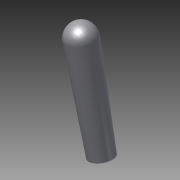
# Autodesk Inventor part: M20S3-toggles
Saved by Autodesk Inventor 2014 (Build 180170000, 170)
## iProperties
Category: PARTsolutions
Company: NKKSWITCHES
Created: 2013-12-29
Part Number: M20S3-toggles
Catalog Web Link: www.cadenas.de
Description: Bushing Mount Miniature Toggles - toggles-Series M - Miniature Toggles
Vendor: NKKSWITCHES
Document SubType Name: Modeling
Designer: PARTuser1
Manufacturer: NKKSWITCHES
Density: 1 g/cm^3
Material: Generic
Appearance: RGB(192.00000375509219,192.00000375509219,192.00000375509219)
PSOL_IDENT_0: {$CADENAS_DATA\23d-libs\nkkswitches\toggle\m\parts\m_bt_toggle.prj},217 {VTYP=3D},{NB=M20S3-toggles}
PSOL_IDENT_1: ,{LINA=M20S3-toggles},{NN=Bushing Mount Miniature Toggles - toggles},{DATE=28.05.2013 12:02:29},{GEO
PSOL_IDENT_2: MDATE=28.05.2013 14:02:00},{VERSION=},{LINEID=10},{LINESUBID=-1},{WBVAR=TGGLS,CPS,CCLR}  {NB=M20S3-t
PSOL_IDENT_3: oggles},{LINA=M20S3-toggles},{KT=DUMMY},{PN=M20S3},{SRS=M20},{TGGLSALG='S', 'S - .413\" (10.5mm) Bat
PSOL_IDENT_4: ','S2', 'S2 - .200\" (5.08mm) Bat','S3', 'S3 - .256\" (6.5mm) Bat','E', 'E - .450\" (11.4mm) Flatted
PSOL_IDENT_5: ','E2', 'E2 - .256\" (6.5mm) Flatted','E4', 'E4 - .840\" (21.3mm) Flatted','Q', 'Q - .550\" (14.0mm)
PSOL_IDENT_6: Cone','Q2', 'Q2 - .640\" (16.26mm) Cone','Q4', 'Q4 - .840\" (21.3mm) Cone','C', 'C - .571\" (14.5mm
PSOL_IDENT_7: ) Color Tipped Cone','D', 'D - .840\" (21.3mm) Color Tipped Cone','K1', 'K1 - .370\" (9.4mm) Paddle'
PSOL_IDENT_8: ,'K2', 'K2 - .559\" (14.2mm) Paddle','B', 'B - .453\" (11.5mm) Large Bat','B2', 'B2 - .689\" (17.5mm
PSOL_IDENT_9: ) Large Bat','R', 'R - .610\" (15.5mm) Large Flatted','L', 'L - .201\" (5.1mm) Dia. Locking Lever'},
PSOL_IDENT_10: {TGGLS=S3},{CPSALG='','N/A'},{CPS=},{CPSPN=},{CCLRALG='','N/A'},{CCLR=},{DSH=},{HEIGHT=0.256},{SHEIG
PSOL_IDENT_11: HT=0.0875},{ROTALG=0.23},{CPCAP=0}
CNS_NN: Bushing Mount Miniature Toggles - toggles
CNS_NT: Series M - Miniature Toggles
CNS_NB: M20S3-toggles
CNS_NBSYN: $PN.-toggles
CNS_LINA: M20S3-toggles
CNS_PN: M20S3
CNS_SRS: M20
CNS_TGGLSALG: 'S', 'S - .413" (10.5mm) Bat','S2', 'S2 - .200" (5.08mm) Bat','S3', 'S3 - .256" (6.5mm) Bat','E', 'E - .450" (11.4mm) Flatted','E2', 'E2 - .256" (6.5mm) Flatted','E4', 'E4 - .840" (21.3mm) Flatted','Q', 'Q - .550" (14.0mm) Cone','Q2', 'Q2 - .640" (16.26mm) Cone','Q4', 'Q4 - .840" (21.3mm) Cone','C', 'C - .571" (14.5mm) Color Tipped Cone','D', 'D - .840" (21.3mm) Color Tipped Cone','K1', 'K1 - .370" (9.4mm) Paddle','K2', 'K2 - .559" (14.2mm) Paddle','B', 'B - .453" (11.5mm) Large Bat','B2', 'B2 - .689" (17.5mm) Large Bat','R', 'R - .610" (15.5mm) Large Flatted','L', 'L - .201" (5.1mm) Dia. Locking Lever'
CNS_TGGLS: S3 - .256" (6.5mm) Bat
CNS_CPSALG: '','N/A'
CNS_CPS: N/A
CNS_CCLRALG: '','N/A'
CNS_CCLR: N/A
CNS_HEIGHT: 0.256
CNS_SHEIGHT: 0.087
CNS_ROTALG: 0.230
CNS_CPCAP: 0.000
SUPPLIER: NKKSWITCHES
ARTICLENO: M20S3-toggles
BOMINFO: M20S3-toggles
CREATOR: CADENAS GmbH
Title: M20S3-toggles
Author: Cadenas PARTsolutions
Comments: Series M - Miniature Toggles
Autodesk Inventor part; units mm, degrees
sketch "Sketch_3" plane through (0, 0, 0) normal (0, 0, 1) x (1, 0, 0)
  line L0 (0.481, -4.3923) -> (-1.9382, 6.5201)
  arc A0 (-0.2719, 5.4586) -> (-1.9382, 6.5201) centre (-1.6358, 5.1562) ccw
  line L1 (-0.2719, 5.4586) -> (1.5949, -4.1454)
  line L2 (1.5949, -4.1454) -> (0.481, -4.3923)
  line L3 (0.481, -4.3923) -> (-1.9382, 6.5201)
  constraints: 8 end point, 2 point on circle, 1 centre point
revolve "Revolution1" add sketch "Sketch_3" angle 360 about axis through (0.481, -4.3923, 0) along (0.2164396, -0.976296, 0)
ref_plane "rot_XY" through (0, -2.2225, 0) normal (0, 0, 1) x (1, 0, 0)
ref_plane "rot_YZ" through (0, -2.2225, 0) normal (1, 0, 0) x (0, 1, 0)
ref_plane "rot_ZX" through (0, -2.2225, 0) normal (0, 1, 0) x (0, 0, 1)
ref_plane "to_cap_XY" through (0, -2.2225, 0) normal (0, 1, 0) x (1, 0, 0)
ref_plane "to_cap_YZ" through (0, -2.2225, 0) normal (1, 0, 0) x (0, 0, -1)
ref_plane "to_cap_ZX" through (0, -2.2225, 0) normal (0, 0, -1) x (0, 1, 0)
body "Solid1"
